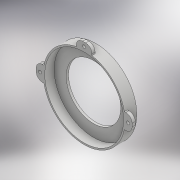
# Autodesk Inventor part: AudioColor
Saved by Autodesk Inventor 2017 (Build 210142000, 142)
## iProperties
Created: 2018-07-23
Part Number: AudioColor
Material: Generic
Document SubType Name: Modeling
Designer: Carolina Lema
Density: 1 g/cm^3
Appearance: Default
Author: Carolina Lema
Autodesk Inventor part; units mm, degrees
ref_plane "YZ Plane" through (0, 0, 0) normal (1, 0, 0) x (0, 1, 0)
ref_plane "XZ Plane" through (0, 0, 0) normal (0, 1, 0) x (-1, 0, 0)
ref_plane "XY Plane" through (0, 0, 0) normal (0, 0, 1) x (1, 0, 0)
sketch "Sketch1" plane through (0, 0, 0) normal (0, 1, 0) x (-1, 0, 0)
  circle A0 centre (0, 0) radius 25.25
  circle A1 centre (0, 0) radius 26.25
  dimension "d0" = 50.5
  dimension "d1" = 52.5
  constraints: 2 centre point, 2 coincident
  measures "d0" diameter of A0
  measures "d1" diameter of A1
extrude "Extrusion1" add sketch "Sketch1" along normal blind 7.5
sketch "Sketch2" plane through (0, 7.5, 0) normal (0, 1, 0) x (1, 0, 0)
  circle A0 centre (0, 0) radius 25.25 projected
  circle A1 centre (0, 0) radius 25.25 projected
  circle A2 centre (0, 0) radius 26.25 projected
  circle A3 centre (0, 0) radius 17.5
  dimension "d4" = 35
  constraints: 1 centre point, 1 coincident
  measures "d4" diameter of A3
extrude "Extrusion2" add sketch "Sketch2" against normal blind 1.5 contours A0
sketch "Sketch3" plane through (0, 0, 0) normal (0, -1, 0) x (1, 0, 0)
  circle A0 centre (0, 0) radius 26.25 projected
  circle A1 centre (0, 0) radius 26.25 projected
  line L0 (26.25, -0.0057) -> (25.75, -0.0057)
  line L1 (-26.25, 0.0058) -> (-25.75, 0.0058)
  line L2 (-0.0095, 26.25) -> (-0.0095, 25.75)
  line L3 (25.75, -0.0057) -> (25.7683, -5.0057)
  line L4 (25.7683, -5.0057) -> (30.7683, -4.9874)
  line L5 (30.7683, -4.9874) -> (30.7317, 5.0125)
  line L6 (30.7317, 5.0125) -> (25.7317, 4.9942)
  line L7 (25.7317, 4.9942) -> (25.7317, 4.9942)
  line L8 (25.75, -0.0057) -> (25.7317, 4.9942)
  line L9 (-0.0095, 25.75) -> (-5.0095, 25.75)
  line L10 (-0.0095, 25.75) -> (4.9905, 25.75) construction
  line L11 (-5.0095, 25.75) -> (-5.0095, 30.75)
  line L12 (-5.0095, 30.75) -> (4.9905, 30.75)
  line L13 (4.9905, 30.75) -> (4.9905, 25.75)
  line L14 (4.9905, 25.75) -> (-0.0095, 25.75)
  line L15 (-25.75, 0.0058) -> (-25.75, -4.9942)
  line L16 (-25.75, 0.0058) -> (-20.75, 0.0058) construction
  line L17 (-25.75, -4.9942) -> (-30.75, -4.9942)
  line L18 (-30.75, -4.9942) -> (-30.75, 5.0058)
  line L19 (-30.75, 5.0058) -> (-25.75, 5.0058)
  line L20 (-25.75, 5.0058) -> (-25.75, 0.0058)
  circle A2 centre (28.2317, 0.0058) radius 1
  circle A3 centre (-28.25, 0.0058) radius 1
  circle A4 centre (-0.0095, 28.25) radius 1
  dimension "d7" = 0.5
  dimension "d8" = 0.5
  dimension "d9" = 0.5
  dimension "d10" = 5
  dimension "d11" = 5
  dimension "d12" = 10
  dimension "d13" = 5
  dimension "d14" = 180
  dimension "d15" = 5
  dimension "d16" = 10
  dimension "d17" = 5
  dimension "d18" = 90
  dimension "d19" = 5
  dimension "d20" = 90
  dimension "d21" = 5
  dimension "d22" = 10
  dimension "d23" = 90
  dimension "d24" = 2
  dimension "d25" = 2
  dimension "d26" = 2
  constraints: 42 end point, 9 perpendicular, 7 point on circle, 5 horizontal, 3 centre point, 2 equal length, 2 point on line, 2 vertical
  measures "d7" distance of L0.start L0.end
  measures "d8" distance of L1.start L1.end
  measures "d9" distance of L2.start L2.end
  measures "d10" distance of L0.end L3.end
  measures "d11" distance of L3.end L4.end
  measures "d12" distance of L4.end L5.end
  measures "d13" distance of L2.end L9.end
  measures "d14" angle of L9 L10
  measures "d15" distance of L9.end L11.end
  measures "d16" distance of L11.end L12.end
  measures "d17" distance of L12.end L13.end
  measures "d18" angle of L12 L13
  measures "d19" distance of L1.end L15.end
  measures "d20" angle of L15 L16
  measures "d21" distance of L15.end L17.end
  measures "d22" distance of L17.end L18.end
  measures "d23" angle of L18 L19
  measures "d24" diameter of A2
  measures "d25" diameter of A3
  measures "d26" diameter of A4
extrude "Extrusion3" add sketch "Sketch3" against normal blind 2 contours A0 L6 L5 L4 | L0 L8 L6 A0 | L17 L18 L19 A0 | A0 L1 L15 L17 | A0 L19 L20 L1 | L13 L14 L2 A0 | A0 L11 L12 L13 | A0 L2 L9 L11
fillet "Fillet1" radius 4 6 edges at (-30.75, 1, -4.9942) (-30.75, 1, 5.0058) (-5.0095, 1, 30.75) (4.9905, 1, 30.75) (30.7317, 1, 5.0125) (30.7683, 1, -4.9874)
body "Solid1"
